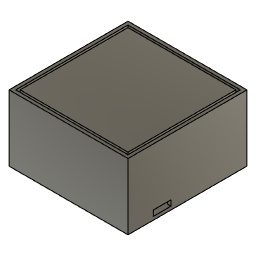
Bomax (Autodesk Fusion 360 design; units mm, degrees)
Autodesk Fusion 360 part; units mm, degrees
sketch "Schizzo1" plane through (0, 0, 0) normal (0, 0, 1) x (1, 0, 0)
  line L0 (0, 0) -> (50, 0)
  line L1 (50, 0) -> (50, 50)
  line L2 (50, 50) -> (0, 50)
  line L3 (0, 50) -> (0, 0)
  line L4 (51.5, -1.5) -> (-1.5, -1.5)
  line L5 (-1.5, -1.5) -> (-1.5, 51.5)
  line L6 (-1.5, 51.5) -> (51.5, 51.5)
  line L7 (51.5, 51.5) -> (51.5, -1.5)
  line L8 (51.5, -1.5) -> (-1.5, 51.5) construction
  line L9 (-1.5, -1.5) -> (51.5, 51.5) construction
  point P0 (25, 25)
  dimension "d1" = 50
  dimension "d2" = 50
  dimension "d4" = 53
  dimension "d5" = 53
  constraint horizontal L0
  constraint vertical L1
  constraint horizontal L2
  constraint vertical L3
  constraint coincident L0.start L3.end
  constraint horizontal L4
  constraint perpendicular L4 L5
  constraint parallel L4 L6
  constraint parallel L5 L7
  constraint coincident L8 P0
  constraint coincident L9 P0
  measures "d1" distance of L0.start L0.end
  measures "d2" distance of L0.start L2.end
  measures "d4" distance of L5.end L6.end
  measures "d5" distance of L4.end L5.end
extrude "Estrusione1" add sketch "Schizzo1" along normal blind 1.5 contours L0 L1 L2 L3 makes body 1
extrude "Estrusione2" add sketch "Schizzo1" along normal blind 25 bodies 1
sketch "Schizzo2" plane through (50, 0, 0) normal (-1, 0, 0) x (0, -1, 0)
  line L0 (-50, 1.5) -> (0, 1.5)
  line L1 (0, 1.5) -> (0, 25)
  line L2 (0, 25) -> (-50, 25)
  line L3 (-50, 25) -> (-50, 1.5)
  line L4 (0, 1.5) -> (-10, 1.5)
  line L5 (-10, 1.5) -> (-10, 4)
  line L6 (-10, 1.5) -> (-18, 1.5)
  line L7 (-18, 1.5) -> (-10, 1.5)
  line L8 (-10, 1.5) -> (-10, 4)
  line L9 (-10, 4) -> (-18, 4)
  line L10 (-18, 4) -> (-18, 1.5)
  dimension "d12" = 10
  dimension "d13" = 2.5
  dimension "d14" = 8
  constraint coincident L0.end L1.start
  constraint perpendicular L1 L4
  constraint perpendicular L0 L5
  constraint perpendicular L5 L6
  constraint horizontal L7
  constraint vertical L8
  constraint horizontal L9
  constraint vertical L10
  measures "d12" distance of L0.end L4.end
  measures "d13" distance of L4.end L5.end
  measures "d14" distance of L4.end L6.end
extrude "Estrusione3" cut sketch "Schizzo2" against normal blind 10 contours L0 L5 L6 L7 L8 L9 L10 bodies 1
sketch "Schizzo4" plane through (0, 0, 1.5) normal (0, 0, 1) x (-1, 0, 0)
  line L0 (0, -50) -> (0, 0)
  line L1 (0, 0) -> (-50, 0)
  line L2 (-50, 0) -> (-50, -10)
  line L3 (-50, -10) -> (-51.5, -10)
  line L4 (-51.5, -10) -> (-51.5, -18)
  line L5 (-51.5, -18) -> (-50, -18)
  line L6 (-50, -18) -> (-50, -50)
  line L7 (-50, -50) -> (0, -50)
  line L8 (-50, 0) -> (-50, -28)
  line L9 (-50, -28) -> (0, -28)
  line L10 (-25, -28) -> (-25, -50)
  line L11 (-28, -42) -> (-22, -42)
  line L12 (-22, -42) -> (-22, -36)
  line L13 (-22, -36) -> (-28, -36)
  line L14 (-28, -36) -> (-28, -42)
  line L15 (-28, -42) -> (-22, -36) construction
  line L16 (-22, -42) -> (-28, -36) construction
  line L17 (-22, -42) -> (-28, -42)
  line L18 (-28, -42) -> (-28, -42.5)
  line L19 (-28, -42.5) -> (-22, -42.5)
  line L20 (-22, -42.5) -> (-22, -42)
  line L21 (-22, -36) -> (-28, -36)
  line L22 (-28, -36) -> (-28, -35.5)
  line L23 (-28, -35.5) -> (-22, -35.5)
  line L24 (-22, -35.5) -> (-22, -36)
  line L25 (-22.5, -40) -> (-21.5, -40)
  line L26 (-21.5, -40) -> (-21.5, -38)
  line L27 (-21.5, -38) -> (-22.5, -38)
  line L28 (-22.5, -38) -> (-22.5, -40)
  line L29 (-22.5, -40) -> (-21.5, -38) construction
  line L30 (-21.5, -40) -> (-22.5, -38) construction
  line L31 (-28.5, -40) -> (-27.5, -40)
  line L32 (-27.5, -40) -> (-27.5, -38)
  line L33 (-27.5, -38) -> (-28.5, -38)
  line L34 (-28.5, -38) -> (-28.5, -40)
  line L35 (-28.5, -40) -> (-27.5, -38) construction
  line L36 (-27.5, -40) -> (-28.5, -38) construction
  point P0 (-25, -39)
  point P1 (-22, -39)
  point P2 (-28, -39)
  dimension "d18" = 28
  dimension "d20" = 6
  dimension "d21" = 6
  dimension "d22" = 0.5
  dimension "d23" = 0.5
  dimension "d24" = 1
  dimension "d25" = 2
  dimension "d26" = 1
  dimension "d27" = 2
  constraint coincident L1.end L2.start
  constraint perpendicular L5 L8
  constraint coincident L0 L9.end
  constraint perpendicular L0 L9
  constraint midpoint L9 L10.start
  constraint midpoint L7 L10.end
  constraint horizontal L11
  constraint perpendicular L11 L12
  constraint parallel L11 L13
  constraint parallel L12 L14
  constraint coincident L15 P0
  constraint coincident L16 P0
  constraint horizontal L17
  constraint vertical L18
  constraint horizontal L19
  constraint vertical L20
  constraint horizontal L21
  constraint vertical L22
  constraint horizontal L23
  constraint vertical L24
  constraint horizontal L25
  constraint perpendicular L25 L26
  constraint parallel L25 L27
  constraint parallel L26 L28
  constraint coincident L29 P1
  constraint coincident L30 P1
  constraint midpoint L12 P1
  constraint horizontal L31
  constraint perpendicular L31 L32
  constraint parallel L31 L33
  constraint parallel L32 L34
  constraint coincident L35 P2
  constraint coincident L36 P2
  constraint midpoint L14 P2
  measures "d18" distance of L1.end L8.end
  measures "d20" distance of L12.end L13.end
  measures "d21" distance of L11.end L12.end
  measures "d22" distance of L11.end L19.end
  measures "d23" distance of L12.end L23.end
  measures "d24" distance of L26.end L27.end
  measures "d25" distance of L25.end L26.end
  measures "d26" distance of L32.end L33.end
  measures "d27" distance of L31.end L32.end
extrude "Estrusione4" add sketch "Schizzo4" along normal blind 12 contours L10 L11 L13 L14 L17 L21 L31 L32 L33 | L10 L11 L12 L13 L17 L21 L25 L27 L28 bodies 1
extrude "Estrusione5" add sketch "Schizzo4" along normal blind 14 contours L10 L11 L17 L18 L19 | L10 L11 L17 L19 L20 | L10 L13 L21 L23 L24 | L10 L13 L21 L22 L23 | L14 L31 L33 L34 | L14 L31 L32 L33 | L12 L25 L27 L28 | L12 L25 L26 L27 bodies 1
extrude "Estrusione6" cut 1 faces at (27.8333, 39.3333, 15.5) along direction (0, 0, -1) blind 2 on bodies 1 bodies 1
extrude "Estrusione7" cut 1 faces at (21.8333, 39.3333, 15.5) along direction (0, 0, -1) blind 2 on bodies 1 bodies 1
extrude "Estrusione8" add sketch "Schizzo4" along normal blind 14 contours L14 L31 L33 L34 | L12 L25 L26 L27 bodies 1
sketch "Schizzo5" plane through (0, 0, 25) normal (0, 0, 1) x (-1, 0, 0)
  line L0 (0, 0) -> (0, -50)
  line L1 (0, -50) -> (-50, -50)
  line L2 (-50, -50) -> (-50, 0)
  line L3 (-50, 0) -> (0, 0)
  line L4 (-51.5, -51.5) -> (1.5, -51.5)
  line L5 (1.5, -51.5) -> (1.5, 1.5)
  line L6 (1.5, 1.5) -> (-51.5, 1.5)
  line L7 (-51.5, 1.5) -> (-51.5, -51.5)
  line L8 (1.5, -51.5) -> (-51.5, -51.5)
  line L9 (-51.5, -51.5) -> (-51.5, 1.5)
  line L10 (-51.5, 1.5) -> (1.5, 1.5)
  line L11 (1.5, 1.5) -> (1.5, -51.5)
  line L12 (0, -50) -> (-50, -50)
  line L13 (-50, -50) -> (-50, 0)
  line L14 (-50, 0) -> (0, 0)
  line L15 (0, 0) -> (0, -50)
  line L16 (-50, 0) -> (-50, -28)
  circle A0 centre (-25, -39) radius 2.5
  line L17 (0, 0) -> (-25, -36.5)
  line L18 (-25, -36.5) -> (-50, 0)
  line L19 (-22.6689, -39.9034) -> (0, 0)
  line L20 (-27.3311, -39.9034) -> (-50, 0)
  line L21 (-22.6689, -39.9034) -> (-25, 0)
  line L22 (-27.3311, -39.9034) -> (-25, 0)
  line L23 (0, -50) -> (-25, -36.5)
  line L24 (0, -50) -> (-25, -41.5)
  line L25 (-25, -41.5) -> (-50, -50)
  line L26 (-25, -36.5) -> (-50, -50)
  dimension "d38" = 28
  dimension "d39" = 5
  constraint horizontal L8
  constraint vertical L9
  constraint horizontal L10
  constraint vertical L11
  constraint coincident L6.end L7.start
  constraint coincident L4.end L5.start
  constraint horizontal L12
  constraint vertical L13
  constraint horizontal L14
  constraint vertical L15
  constraint coincident L2.end L3.start
  constraint coincident L0.end L1.start
  constraint perpendicular L14 L16
  constraint coincident L0.start L3.end
  constraint coincident A0 L17.end
  constraint coincident A0 L19.start
  constraint coincident A0 L20.start
  constraint midpoint L14 L21.end
  constraint coincident A0 L24.end
  constraint coincident L1.end L2.start
  measures "d38" distance of L2.end L16.end
  measures "d39" diameter of A0
extrude "Estrusione9" add sketch "Schizzo5" against normal blind 6.5 separate body contours A0 L21 L22 L23 L26 | A0 L26 | A0 L23 | A0 L21 | A0 L22 makes body 2
extrude "Estrusione10" add sketch "Schizzo5" along normal blind 5 bodies 1
extrude "Estrusione11" add sketch "Schizzo5" along normal blind 5 contours L3 L14 L17 L21 | L17 L19 L21 L23 | L0 L15 L19 L23 | A0 L19 L23 L24 | L1 L12 L24 L25 | L3 L14 L18 L22 | L17 L18 L21 L22 | A0 L17 L21 L23 | A0 L19 L21 L23 | A0 L20 L25 L26 | L2 L13 L16 L20 L26 | A0 L21 L22 L23 L26 | L18 L20 L22 L26 | A0 L18 L22 L26 | A0 L26 | A0 L23 | A0 L21 L23 | A0 L21 | A0 L20 L22 L26 | A0 L22 | A0 L22 L26 bodies 2
sketch "Schizzo7" plane through (50, 0, 0) normal (1, 0, 0) x (0, 1, 0)
  line L0 (0, 25) -> (50, 25)
  line L1 (50, 25) -> (50, 30)
  line L2 (50, 30) -> (0, 30)
  line L3 (0, 30) -> (0, 25)
  line L4 (0, 30) -> (50, 30)
  line L5 (50, 30) -> (50, 25)
  line L6 (50, 25) -> (0, 25)
  line L7 (0, 25) -> (0, 30)
  line L8 (28, 25) -> (50, 25)
  line L9 (39, 25) -> (39, 18.5)
  line L10 (39, 18.5) -> (39, 20.5)
  line L11 (39, 20.5) -> (0, 25)
  line L12 (39, 20.5) -> (50, 25)
  dimension "d46" = 28
  dimension "d47" = 6.5
  dimension "d48" = 2
  constraint horizontal L4
  constraint vertical L5
  constraint horizontal L6
  constraint vertical L7
  constraint coincident L0.end L1.start
  constraint coincident L2.end L3.start
  constraint midpoint L8 L9.start
  constraint perpendicular L6 L9
  constraint perpendicular L6 L10
  constraint coincident L0.start L3.end
  measures "d46" distance of L0.start L8.start
  measures "d47" distance of L9.start L9.end
  measures "d48" distance of L9.end L10.end
extrude "Estrusione12" add sketch "Schizzo7" against normal blind 50 contours L0 L6 L8 L9 L11 | L0 L6 L8 L9 L12 bodies 2
sketch "Schizzo8" plane through (0, 0, 0) normal (0, -1, 0) x (1, 0, 0)
  line L0 (0, 25) -> (50, 25)
  line L1 (50, 25) -> (50, 30)
  line L2 (50, 30) -> (0, 30)
  line L3 (0, 30) -> (0, 25)
  line L4 (0, 30) -> (50, 30)
  line L5 (50, 30) -> (50, 25)
  line L6 (50, 25) -> (0, 25)
  line L7 (0, 25) -> (0, 30)
  line L8 (25, 25) -> (25, 18.5)
  line L9 (25, 18.5) -> (25, 20.5)
  line L10 (25, 20.5) -> (50, 25)
  line L11 (25, 20.5) -> (0, 25)
  line L12 (0, 25) -> (0, 20.5)
  line L13 (0, 20.5) -> (25, 20.5)
  line L14 (25, 20.5) -> (50, 20.5)
  line L15 (50, 20.5) -> (50, 25)
  dimension "d51" = 6.5
  dimension "d52" = 2
  constraint horizontal L4
  constraint vertical L5
  constraint horizontal L6
  constraint vertical L7
  constraint coincident L0.end L1.start
  constraint coincident L2.end L3.start
  constraint midpoint L6 L8.start
  constraint perpendicular L6 L8
  constraint perpendicular L6 L9
  constraint coincident L0.start L3.end
  constraint perpendicular L6 L12
  constraint perpendicular L9 L13
  constraint perpendicular L1 L14
  constraint perpendicular L6 L15
  measures "d51" distance of L8.start L8.end
  measures "d52" distance of L8.end L9.end
extrude "Estrusione13" cut sketch "Schizzo8" against normal blind 71 contours L11 L12 L13 | L10 L14 L15 bodies 2
extrude "Estrusione14" add 1 faces at (24.2037, 39.4775, 18.5) along direction (0, 0, 1) blind 5 on bodies 2 bodies 2
extrude "Estrusione15" cut 1 faces at (33.3333, 0, 26.6667) along direction (0, 1, 0) blind 0.5 on bodies 2 bodies 2
extrude "Estrusione16" cut 1 faces at (33.3333, 0.3333, 25) along direction (0, 0, -1) blind 8 on bodies 2 bodies 2
extrude "Estrusione17" cut 1 faces at (50, 17, 28.3333) along direction (-1, 0, 0) blind 0.5 on bodies 2 bodies 2
extrude "Estrusione18" cut 1 faces at (49.8333, 17, 25) along direction (0, 0, -1) blind 10 on bodies 2 bodies 2
extrude "Estrusione19" cut 1 faces at (16.5, 50, 26.6667) along direction (0, -1, 0) blind 0.5 on bodies 2 bodies 2
extrude "Estrusione20" cut 1 faces at (16.5, 49.8333, 25) along direction (0, 0, -1) blind 4 on bodies 2 bodies 2
extrude "Estrusione21" cut 1 faces at (0, 16.8333, 28.3333) along direction (1, 0, 0) blind 0.5 on bodies 2 bodies 2
extrude "Estrusione22" cut 1 faces at (0.1667, 16.8333, 25) along direction (0, 0, -1) blind 6 on bodies 2 bodies 2
extrude "Estrusione23" cut 1 faces at (0, 16.6667, 20.5) along direction (-1, 0, 0) blind 0.5 on bodies 1 bodies 1
extrude "Estrusione24" cut 1 faces at (16.3333, 50, 11) along direction (0, 1, 0) blind 0.5 on bodies 1 bodies 1
extrude "Estrusione25" add 1 faces at (33.8333, 51.5, 20) along direction (0, 1, 0) blind 0.5 on bodies 1 bodies 1
extrude "Estrusione26" add 1 faces at (-1.5, 34.1667, 10) along direction (-1, 0, 0) blind 0.5 on bodies 1 bodies 1
extrude "Estrusione27" cut 1 faces at (50, 22.8333, 21.3333) along direction (1, 0, 0) blind 0.5 on bodies 1 bodies 1
extrude "Estrusione28" cut 1 faces at (33.5, 0, 11) along direction (0, -1, 0) blind 0.5 on bodies 1 bodies 1
extrude "Estrusione29" add 1 faces at (15.8333, -1.5, 10) along direction (0, -1, 0) blind 0.5 on bodies 1 bodies 1
extrude "Estrusione30" add 1 faces at (51.5, 22.6667, 21.3333) along direction (1, 0, 0) blind 0.5 on bodies 1 bodies 1
extrude "Estrusione31" cut 1 faces at (51.5, 10, 2.3333) along direction (0, -1, 0) blind 0.5 on bodies 1 bodies 1
extrude "Estrusione32" add 1 faces at (51, 18, 2.3333) along direction (0, -1, 0) blind 0.5 on bodies 1 bodies 1
sketch "Schizzo9" plane through (0, 0, 1.5) normal (0, 0, 1) x (-1, 0, 0)
  line L0 (-50.5, -17.5) -> (-50.5, -50.5)
  line L1 (-50.5, -50.5) -> (0.5, -50.5)
  line L2 (0.5, -50.5) -> (0.5, 0.5)
  line L3 (0.5, 0.5) -> (-50.5, 0.5)
  line L4 (-50.5, 0.5) -> (-50.5, -9.5)
  line L5 (-50.5, -9.5) -> (-52, -9.5)
  line L6 (-52, -9.5) -> (-52, -17.5)
  line L7 (-52, -17.5) -> (-50.5, -17.5)
  line L8 (-28, -42.5) -> (-28, -40)
  line L9 (-28, -40) -> (-28.5, -40)
  line L10 (-28.5, -40) -> (-28.5, -38)
  line L11 (-28.5, -38) -> (-28, -38)
  line L12 (-28, -38) -> (-28, -35.5)
  line L13 (-28, -35.5) -> (-22, -35.5)
  line L14 (-22, -35.5) -> (-22, -38)
  line L15 (-22, -38) -> (-21.5, -38)
  line L16 (-21.5, -38) -> (-21.5, -40)
  line L17 (-21.5, -40) -> (-22, -40)
  line L18 (-22, -40) -> (-22, -42.5)
  line L19 (-22, -42.5) -> (-28, -42.5)
  line L20 (-50.5, 0.5) -> (-50.5, -27.5)
  line L21 (-50.5, -27.5) -> (0.5, -27.5)
  line L22 (0.5, 0.5) -> (-0.5, 0.5)
  line L23 (-0.5, 0.5) -> (-0.5, -27.5)
  line L24 (0.5, -27.5) -> (0.5, -28.5)
  line L25 (0.5, -28.5) -> (-50.5, -28.5)
  dimension "d93" = 28
  dimension "d94" = 1
  dimension "d95" = 1
  constraint coincident L3.end L4.start
  constraint perpendicular L7 L20
  constraint coincident L2 L21.end
  constraint perpendicular L2 L21
  constraint coincident L2.end L3.start
  constraint perpendicular L2 L22
  constraint coincident L21 L23.end
  constraint perpendicular L21 L23
  constraint coincident L0 L25.end
  constraint perpendicular L0 L25
  measures "d93" distance of L3.end L20.end
  measures "d94" distance of L2.end L22.end
  measures "d95" distance of L21.end L24.end
extrude "Estrusione33" add sketch "Schizzo9" along normal blind 6 contours L0 L2 L21 L24 L25 | L2 L3 L21 L22 L23 bodies 1
